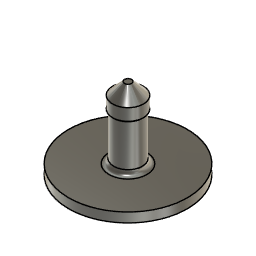
Alfa 147 Hatch Bolt v2 (Autodesk Fusion 360 design; units mm, degrees)
Autodesk Fusion 360 part; units mm, degrees
sketch "Sketch1" plane through (0, 0, 0) normal (0, 0, 1) x (1, 0, 0)
  circle A0 centre (0, 0) radius 12.5
  constraint coincident A0.centre origin
extrude "Extrude1" add sketch "Sketch1" along normal blind 2
sketch "Sketch2" plane through (0, 0, 2) normal (0, 0, 1) x (-1, 0, 0)
  circle A0 centre (0, 0) radius 12.5
  circle A1 centre (0, 0) radius 3
  constraint coincident A0.centre A1.centre
extrude "Extrude2" add sketch "Sketch2" along normal blind 10 contours A1
sketch "Sketch3" plane through (0, 0, 12) normal (0, 0, 1) x (-1, 0, 0)
  circle A0 centre (0, 0) radius 3
  circle A1 centre (0, 0) radius 3.25
  dimension "d8" = 6.5
  constraint coincident A0.centre A1.centre
  measures "d8" diameter of A1
extrude "Extrude3" add sketch "Sketch3" along normal blind 5 contours A0 | A1
chamfer "Chamfer1" distance 2.5 angle 45 1 edges at (3.0301, 1.1753, 17)
chamfer "Chamfer2" distance 0.25 angle 45 1 edges at (2.797, 1.0848, 12)
fillet "Fillet1" radius 1 1 edges at (2.797, -1.0848, 2)
